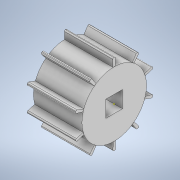
# Autodesk Inventor part: 220411 Large Rod Laddered
Saved by Autodesk Inventor 2022 (Build 260153000, 153)
## iProperties
Created: 2022-01-22
Part Number: 220411 Large Rod Laddered
Material: Generic
Document SubType Name: Modeling
Designer: josephinew
Density: 1 g/cm^3
Appearance: Default
Author: josephinew
Autodesk Inventor part; units mm, degrees
ref_plane "YZ Plane" through (0, 0, 0) normal (1, 0, 0) x (0, 1, 0)
ref_plane "XZ Plane" through (0, 0, 0) normal (0, 1, 0) x (-1, 0, 0)
ref_plane "XY Plane" through (0, 0, 0) normal (0, 0, 1) x (1, 0, 0)
sketch "Sketch1" plane through (0, 0, 0) normal (1, 0, 0) x (0, 1, 0)
  circle A0 centre (-0.127, -0.127) radius 50.8
  line L0 (13.081, 13.081) -> (-13.081, 13.081)
  line L1 (-13.081, 13.081) -> (-13.081, -13.081)
  line L2 (-13.081, -13.081) -> (13.081, -13.081)
  line L3 (13.081, -13.081) -> (13.081, 13.081)
  dimension "d58" = 26.162
  dimension "d59" = 26.162
  constraints: 8 end point, 2 parallel, 1 centre point, 1 horizontal, 1 perpendicular
  measures "d58" distance of L2.end L1.end
  measures "d59" distance of L1.end L0.end
extrude "Extrusion1" add sketch "Sketch1" along normal blind 76.2
sketch "Sketch4" plane through (76.2, 0, 0) normal (1, 0, 0) x (0, 0, -1)
  line L0 (0, 0) -> (62.0637, 0) construction
  line L1 (0, 0) -> (66.7156, 0) construction
  line L2 (0, 0) -> (71.481, 0) construction
  line L3 (0, 0) -> (54.0079, 0) construction
  line L4 (0, 0) -> (54.0079, 0) construction
  line L5 (1.7729, 50.7691) -> (1.9647, 56.2627)
  line L6 (0, 0) -> (63.5387, 0) construction
  line L7 (-1.7729, 50.7691) -> (-1.9647, 56.2627)
  line L8 (0, 0) -> (61.9502, 0) construction
  arc A0 (0.5882, 63.4973) -> (-0.5882, 63.4973) centre (0, 0) ccw
  line L9 (1.7729, 50.7691) -> (2.16, 61.8544)
  line L10 (-1.7729, 50.7691) -> (-2.16, 61.8544)
  arc A1 (-0.5882, 63.4973) -> (-2.16, 61.8544) centre (-0.5735, 61.9098) ccw
  arc A2 (2.16, 61.8544) -> (0.5882, 63.4973) centre (0.5735, 61.9098) ccw
  circle A3 centre (0, 0) radius 50.8
  point P0 (1.9945, 57.1152)
  point P1 (-1.9945, 57.1152)
  point P2 (2.2161, 63.4613)
  point P3 (-2.2161, 63.4613)
  dimension "d52" = 127
  dimension "d53" = 1.5875
  constraints: 22 end point, 8 point on circle, 7 horizontal, 4 point on line, 4 tangent, 3 centre point, 3 coincident, 1 equal radius, 3 other
  measures "d52" diameter of A0
  measures "d53" radius of A1
extrude "Extrusion4" add sketch "Sketch4" against normal blind 76.2 contours A3 L7 L10 A1 A0 A2 L9 L5
pattern_circular "Circular Pattern2" count 10 over 360 about axis through (0, -0.127, -0.127) along (1, 0, 0) of "Extrusion4"
sketch "Sketch5" plane through (76.2, -0.127, -0.127) normal (1, 0, 0) x (0, 0, -1)
  point P0 (-0.127, 0.127)
body "Solid1"
